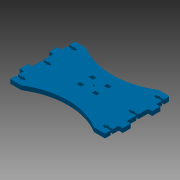
# Autodesk Inventor part: czesc6
Saved by Autodesk Inventor 2013 (Build 170138000, 138)
## iProperties
Created: 2014-01-17
Part Number: czesc6
Material: Generic
Document SubType Name: Modeling
Designer: dzban
Density: 1 g/cm^3
Author: dzban
Autodesk Inventor part; units mm, degrees
ref_plane "YZ Plane" through (0, 0, 0) normal (1, 0, 0) x (0, 1, 0)
ref_plane "XZ Plane" through (0, 0, 0) normal (0, 1, 0) x (-1, 0, 0)
ref_plane "XY Plane" through (0, 0, 0) normal (0, 0, 1) x (1, 0, 0)
sketch "Sketch1" plane through (0, 0, 0) normal (0, 0, 1) x (1, 0, 0)
  line L0 (19.6928, -26.0637) -> (19.6928, -36.0637)
  line L1 (19.6928, -36.0637) -> (83.1928, -36.0637)
  line L2 (83.1928, -36.0637) -> (83.1928, -27.5637)
  line L3 (83.1928, -27.5637) -> (76.1894, -27.5637)
  line L4 (76.1894, -27.5637) -> (76.1894, -28.8137)
  line L5 (76.1894, -28.8137) -> (74.3894, -28.8137)
  line L6 (74.3894, -28.8137) -> (74.3894, -27.5637)
  line L7 (74.3894, -27.5637) -> (71.3894, -27.5637)
  line L8 (71.3894, -27.5637) -> (71.3894, -24.5637)
  line L9 (71.3894, -24.5637) -> (74.3894, -24.5637)
  line L10 (74.3894, -24.5637) -> (74.3894, -23.3137)
  line L11 (74.3894, -23.3137) -> (76.1894, -23.3137)
  line L12 (76.1894, -23.3137) -> (76.1894, -24.5637)
  line L13 (76.1894, -24.5637) -> (83.1928, -24.5637)
  line L14 (83.1928, -24.5637) -> (83.1928, -16.1637)
  line L15 (83.1928, -16.1637) -> (89.1928, -16.0637)
  line L16 (89.1928, -16.0637) -> (89.1928, -4.2637)
  line L17 (89.1928, -4.2637) -> (83.1928, -4.1637)
  line L18 (83.1928, -4.1637) -> (83.1928, 9.9363)
  line L19 (83.1928, 9.9363) -> (76.1894, 9.9363)
  line L20 (76.1894, 9.9363) -> (76.1894, 8.6863)
  line L21 (76.1894, 8.6863) -> (74.3894, 8.6863)
  line L22 (74.3894, 8.6863) -> (74.3894, 9.9363)
  line L23 (74.3894, 9.9363) -> (71.3894, 9.9363)
  line L24 (71.3894, 9.9363) -> (71.3894, 12.9363)
  line L25 (71.3894, 12.9363) -> (74.3894, 12.9363)
  line L26 (74.3894, 12.9363) -> (74.3894, 14.1863)
  line L27 (74.3894, 14.1863) -> (76.1894, 14.1863)
  line L28 (76.1894, 14.1863) -> (76.1894, 12.9363)
  line L29 (76.1894, 12.9363) -> (83.1928, 12.9363)
  line L30 (83.1928, 12.9363) -> (83.1928, 27.0363)
  line L31 (83.1928, 27.0363) -> (89.1928, 27.1363)
  line L32 (89.1928, 27.1363) -> (89.1928, 38.9363)
  line L33 (89.1928, 38.9363) -> (83.1928, 39.0363)
  line L34 (83.1928, 39.0363) -> (83.1928, 47.4363)
  line L35 (83.1928, 47.4363) -> (76.1894, 47.4363)
  line L36 (76.1894, 47.4363) -> (76.1894, 46.1863)
  line L37 (76.1894, 46.1863) -> (74.3894, 46.1863)
  line L38 (74.3894, 46.1863) -> (74.3894, 47.4363)
  line L39 (74.3894, 47.4363) -> (71.3894, 47.4363)
  line L40 (71.3894, 47.4363) -> (71.3894, 50.4363)
  line L41 (71.3894, 50.4363) -> (74.3894, 50.4363)
  line L42 (74.3894, 50.4363) -> (74.3894, 51.6863)
  line L43 (74.3894, 51.6863) -> (76.1894, 51.6863)
  line L44 (76.1894, 51.6863) -> (76.1894, 50.4363)
  line L45 (76.1894, 50.4363) -> (83.1928, 50.4363)
  line L46 (83.1928, 50.4363) -> (83.1928, 52.9373)
  line L47 (83.1928, 55.937) -> (83.1928, 56.9363)
  arc A0 (83.1928, 56.9363) -> (81.1928, 58.9363) centre (81.1928, 56.9363) ccw
  line L48 (81.1928, 58.9363) -> (-53.8072, 58.9363)
  arc A1 (-53.8072, 58.9363) -> (-55.8072, 56.9363) centre (-53.8072, 56.9363) ccw
  line L49 (-55.8072, 56.9363) -> (-55.8072, 55.9363)
  line L50 (-55.8072, 52.9363) -> (-55.8072, 50.4363)
  line L51 (-55.8072, 50.4363) -> (-48.8072, 50.4363)
  line L52 (-48.8072, 50.4363) -> (-48.8072, 51.6863)
  line L53 (-48.8072, 51.6863) -> (-47.0072, 51.6863)
  line L54 (-47.0072, 51.6863) -> (-47.0072, 50.4363)
  line L55 (-47.0072, 50.4363) -> (-44.0716, 50.4363)
  line L56 (-44.0716, 50.4363) -> (-44.0716, 47.4363)
  line L57 (-44.0716, 47.4363) -> (-47.0072, 47.4363)
  line L58 (-47.0072, 47.4363) -> (-47.0072, 46.1863)
  line L59 (-47.0072, 46.1863) -> (-48.8072, 46.1863)
  line L60 (-48.8072, 46.1863) -> (-48.8072, 47.4363)
  line L61 (-48.8072, 47.4363) -> (-55.8072, 47.4363)
  line L62 (-55.8072, 47.4363) -> (-55.8072, 39.0363)
  line L63 (-55.8072, 39.0363) -> (-61.8072, 38.9363)
  line L64 (-61.8072, 38.9363) -> (-61.8072, 27.1363)
  line L65 (-61.8072, 27.1363) -> (-55.8072, 27.0363)
  line L66 (-55.8072, 27.0363) -> (-55.8072, 12.9363)
  line L67 (-55.8072, 12.9363) -> (-48.8072, 12.9363)
  line L68 (-48.8072, 12.9363) -> (-48.8072, 14.1863)
  line L69 (-48.8072, 14.1863) -> (-47.0072, 14.1863)
  line L70 (-47.0072, 14.1863) -> (-47.0072, 12.9363)
  line L71 (-47.0072, 12.9363) -> (-44.0716, 12.9363)
  line L72 (-44.0716, 12.9363) -> (-44.0716, 9.9363)
  line L73 (-44.0716, 9.9363) -> (-47.0072, 9.9363)
  line L74 (-47.0072, 9.9363) -> (-47.0072, 8.6863)
  line L75 (-47.0072, 8.6863) -> (-48.8072, 8.6863)
  line L76 (-48.8072, 8.6863) -> (-48.8072, 9.9363)
  line L77 (-48.8072, 9.9363) -> (-55.8072, 9.9363)
  line L78 (-55.8072, 9.9363) -> (-55.8072, -4.1637)
  line L79 (-55.8072, -4.1637) -> (-61.8072, -4.2637)
  line L80 (-61.8072, -4.2637) -> (-61.8072, -16.0637)
  line L81 (-61.8072, -16.0637) -> (-55.8072, -16.1637)
  line L82 (-55.8072, -16.1637) -> (-55.8072, -24.5637)
  line L83 (-55.8072, -24.5637) -> (-48.8072, -24.5637)
  line L84 (-48.8072, -24.5637) -> (-48.8072, -23.3137)
  line L85 (-48.8072, -23.3137) -> (-47.0072, -23.3137)
  line L86 (-47.0072, -23.3137) -> (-47.0072, -24.5637)
  line L87 (-47.0072, -24.5637) -> (-44.0716, -24.5637)
  line L88 (-44.0716, -24.5637) -> (-44.0716, -27.5637)
  line L89 (-44.0716, -27.5637) -> (-47.0072, -27.5637)
  line L90 (-47.0072, -27.5637) -> (-47.0072, -28.8137)
  line L91 (-47.0072, -28.8137) -> (-48.8072, -28.8137)
  line L92 (-48.8072, -28.8137) -> (-48.8072, -27.5637)
  line L93 (-48.8072, -27.5637) -> (-55.8072, -27.5637)
  line L94 (-55.8072, -27.5637) -> (-55.8072, -36.0637)
  line L95 (-55.8072, -36.0637) -> (7.6928, -36.0637)
  line L96 (7.6928, -36.0637) -> (7.6928, -26.0637)
  line L97 (7.6928, -26.0637) -> (19.6928, -26.0637)
  line L98 (5.6928, 6.2364) -> (-0.7072, 6.2364)
  line L99 (-0.7072, 6.2364) -> (-0.7072, 11.2364)
  line L100 (-0.7072, 11.2364) -> (5.6928, 11.2364)
  line L101 (5.6928, 11.2364) -> (5.6928, 6.2364)
  line L102 (28.0928, 6.2364) -> (21.6928, 6.2364)
  line L103 (21.6928, 6.2364) -> (21.6928, 11.2364)
  line L104 (21.6928, 11.2364) -> (28.0928, 11.2364)
  line L105 (28.0928, 11.2364) -> (28.0928, 6.2364)
  line L106 (28.0928, 23.8364) -> (21.6928, 23.8364)
  line L107 (21.6928, 23.8364) -> (21.6928, 28.8364)
  line L108 (21.6928, 28.8364) -> (28.0928, 28.8364)
  line L109 (28.0928, 28.8364) -> (28.0928, 23.8364)
  line L110 (5.6928, 28.8364) -> (5.6928, 23.8364)
  line L111 (5.6928, 23.8364) -> (-0.7072, 23.8364)
  line L112 (-0.7072, 23.8364) -> (-0.7072, 28.8364)
  line L113 (-0.7072, 28.8364) -> (5.6928, 28.8364)
  line L114 (-55.8072, 52.9363) -> (-55.8072, 55.9363)
  line L115 (83.1928, 52.9373) -> (83.1928, 55.937)
  circle A2 centre (13.6928, 17.2364) radius 1
  point P0 (0, 0)
  dimension "d0" = 58.9363
  dimension "d1" = 139
  dimension "d2" = 95
  dimension "d3" = 55.8072
  dimension "d4" = 6
  dimension "d5" = 2
  dimension "d6" = 12
  dimension "d7" = 12
  dimension "d8" = 11.7356
  dimension "d9" = 2.9356
  dimension "d10" = 1.8
  dimension "d11" = 3
  dimension "d12" = 1.25
  dimension "d13" = 1.25
  dimension "d14" = 8.5
  dimension "d15" = 3
  dimension "d16" = 1.25
  dimension "d17" = 1.25
  dimension "d18" = 8.5
  dimension "d19" = 19.9
  dimension "d20" = 0.1
  dimension "d21" = 11.8
  dimension "d22" = 46
  dimension "d23" = 3
  dimension "d24" = 1.25
  dimension "d25" = 1.25
  dimension "d26" = 19.9
  dimension "d27" = 6.4
  dimension "d28" = 5
  dimension "d29" = 6.4
  dimension "d30" = 5
  dimension "d31" = 12.6
  dimension "d32" = 16
  dimension "d33" = 30.1
  dimension "d34" = 55.1
  dimension "d35" = 11.8033
  dimension "d36" = 3
  dimension "d37" = 1.8
  dimension "d38" = 6
  dimension "d39" = 12
  dimension "d40" = 10
  dimension "d41" = 63.5
  dimension "d43" = 2
  dimension "d44" = 8
  dimension "d45" = 6.6
  constraints: 232 end point, 82 parallel, 63 collinear, 22 perpendicular, 16 tangent, 4 horizontal alignment, 4 point on circle, 3 centre point, 1 equal radius, 1 horizontal
  measures "d0" distance from line of L48 point (0, 0)
  measures "d1" distance between parallel lines of L47 L49
  measures "d2" distance between parallel lines of L48 L95
  measures "d3" distance from line of L49 point (0, 0)
  measures "d4" distance between parallel lines of L94 L80
  measures "d5" radius of A1
  measures "d6" distance of L62.end L65.end
  measures "d7" distance of L78.end L82.start
  measures "d8" distance between parallel lines of L50 L56
  measures "d9" distance between parallel lines of L56 L54
  measures "d10" distance between parallel lines of L54 L52
  measures "d11" distance between parallel lines of L51 L61
  measures "d12" distance between parallel lines of L53 L51
  measures "d13" distance from line of L57 L59.start
  measures "d14" distance between parallel lines of L48 L51
  measures "d15" distance between parallel lines of L83 L93
  measures "d16" distance between parallel lines of L89 L91
  measures "d17" distance between parallel lines of L85 L87
  measures "d18" distance between parallel lines of L93 L95
  measures "d19" distance from line of L48 L62.end
  measures "d20" vertical distance of L62.end L63.end
  measures "d21" distance of L63.end L65.start
  measures "d22" distance between parallel lines of L77 L95
  measures "d23" distance between parallel lines of L67 L77
  measures "d24" distance between parallel lines of L73 L75
  measures "d25" distance between parallel lines of L71 L69
  measures "d26" distance from line of L82.start L95
  measures "d27" distance between parallel lines of L110 L112
  measures "d28" distance between parallel lines of L113 L111
  measures "d29" distance between parallel lines of L109 L107
  measures "d30" distance between parallel lines of L100 L98
  measures "d31" distance between parallel lines of L111 L100
  measures "d32" distance between parallel lines of L107 L110
  measures "d33" distance between parallel lines of L48 L113
  measures "d34" distance between parallel lines of L112 L66
  measures "d35" distance between parallel lines of L46 L40
  measures "d36" distance between parallel lines of L42 L40
  measures "d37" distance between parallel lines of L44 L42
  measures "d38" distance from line of L115.end L32
  measures "d39" distance between parallel lines of L0 L96
  measures "d40" distance between parallel lines of L97 L1
  measures "d41" distance between parallel lines of L96 L94
  measures "d43" diameter of A2
  measures "d44" distance from line of L107 A2.centre
  measures "d45" distance from line of L106 A2.centre
extrude "Extrusion1" add sketch "Sketch1" along normal blind 6
sketch "Sketch2" plane through (0, 0, 0) normal (0, 0, -1) x (-1, 0, 0)
  circle A0 centre (-13.6928, 17.2364) radius 1 projected
  circle A1 centre (-13.6928, -122.5171) radius 101.5933
  line L0 (-7.6928, -36.0637) -> (55.8072, -36.0637) projected
  line L1 (107.5733, 11.4363) -> (218.4017, 11.4363) construction
  circle A2 centre (-13.6928, 145.3898) radius 101.5933
  line L2 (53.8072, 58.9363) -> (-81.1928, 58.9363) projected
  point P0 (0, 0)
  dimension "d50" = 47.5
  dimension "d51" = 203.1866
  dimension "d52" = 86.4535
  constraints: 2 centre point, 2 end point, 1 horizontal, 1 symmetric about line, 1 vertical alignment, 1 other
  measures "d50" distance between parallel lines of L1 L0
  measures "d51" diameter of A1
  measures "d52" distance from line of L2 A2.centre
extrude "Extrusion2" cut sketch "Sketch2" against normal blind 10 contours A1 | A2 L2 | L2 A2
body "Solid1"
